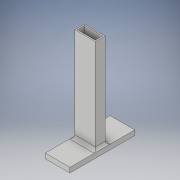
# Autodesk Inventor part: Pizza1
Saved by Autodesk Inventor 2018.2 (Build 222227000, 227)
## iProperties
Created: 2018-03-29
Part Number: Pizza1
Material: Generic
Document SubType Name: Modeling
Designer: MIABo
Density: 1 g/cm^3
Appearance: Default
Author: MIABo
Autodesk Inventor part; units mm, degrees
ref_plane "YZ Plane" through (0, 0, 0) normal (1, 0, 0) x (0, 1, 0)
ref_plane "XZ Plane" through (0, 0, 0) normal (0, 1, 0) x (-1, 0, 0)
ref_plane "XY Plane" through (0, 0, 0) normal (0, 0, 1) x (1, 0, 0)
sketch "Sketch1" plane through (0, 0, 0) normal (0, 1, 0) x (-1, 0, 0)
  line L0 (12.7, 33.3375) -> (-12.7, 33.3375)
  line L1 (-12.7, 33.3375) -> (-12.7, -33.3375)
  line L2 (-12.7, -33.3375) -> (12.7, -33.3375)
  line L3 (12.7, -33.3375) -> (12.7, 33.3375)
  line L4 (12.7, 33.3375) -> (-12.7, -33.3375) construction
  line L5 (-12.7, 33.3375) -> (12.7, -33.3375) construction
  point P0 (0, 0)
  dimension "d0" = 25.4
  dimension "d1" = 66.675
  constraints: 12 end point, 2 midpoint, 2 parallel, 1 horizontal, 1 perpendicular
  measures "d0" distance of L2.end L1.end
  measures "d1" distance of L1.end L0.end
extrude "Extrusion1" add sketch "Sketch1" along normal blind 5.08
sketch "Sketch3" plane through (0, 5.08, 0) normal (0, 1, 0) x (1, 0, 0)
  line L0 (-10.541, 5.08) -> (10.541, 5.08)
  line L1 (10.541, 5.08) -> (10.541, -5.08)
  line L2 (10.541, -5.08) -> (-10.541, -5.08)
  line L3 (-10.541, -5.08) -> (-10.541, 5.08)
  line L4 (-10.541, 5.08) -> (10.541, -5.08) construction
  line L5 (10.541, 5.08) -> (-10.541, -5.08) construction
  point P0 (0, 0)
  dimension "d8" = 21.082
  dimension "d9" = 10.16
  constraints: 12 end point, 2 midpoint, 2 parallel, 1 horizontal, 1 perpendicular
  measures "d8" distance of L1.end L2.end
  measures "d9" distance of L0.end L1.end
extrude "Extrusion3" add sketch "Sketch3" along normal blind 96.8375
sketch "Sketch2" plane through (0, 5.08, 0) normal (0, 1, 0) x (1, 0, 0)
  line L0 (-9.271, -3.81) -> (9.271, -3.81)
  line L1 (9.271, -3.81) -> (9.271, 3.81)
  line L2 (9.271, 3.81) -> (-9.271, 3.81)
  line L3 (-9.271, 3.81) -> (-9.271, -3.81)
  line L4 (-9.271, -3.81) -> (9.271, 3.81) construction
  line L5 (9.271, -3.81) -> (-9.271, 3.81) construction
  point P0 (0, 0)
  dimension "d4" = 18.542
  dimension "d5" = 7.62
  constraints: 12 end point, 2 midpoint, 2 parallel, 1 horizontal, 1 perpendicular
  measures "d4" distance of L2.end L1.end
  measures "d5" distance of L1.end L0.end
extrude "Extrusion2" cut sketch "Sketch2" along normal through all both and the other way through all
fillet "Fillet1" radius 3.175 4 edges at (0, 5.08, 5.08) (10.541, 5.08, 0) (0, 5.08, -5.08) (-10.541, 5.08, 0)
body "Solid1"
